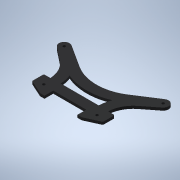
# Autodesk Inventor part: back_plate
Saved by Autodesk Inventor 2020 (Build 240168000, 168)
## iProperties
Created: 2016-01-08
Part Number: back_plate
Material: Genérico
Document SubType Name: Modeling
Designer: MIGUEL ANGEL
Density: 1 g/cm^3
Appearance: Goma - Negro
Author: MIGUEL ANGEL
Autodesk Inventor part; units mm, degrees
ref_plane "YZ Plane" through (0, 0, 0) normal (1, 0, 0) x (0, 1, 0)
ref_plane "XZ Plane" through (0, 0, 0) normal (0, 1, 0) x (-1, 0, 0)
sketch "Boceto1" plane through (0, 0, 0) normal (0, 0, 1) x (1, 0, 0)
  line L0 (20.4772, 24.8969) -> (57.9772, 24.8969)
  line L1 (86.0741, 43.5717) -> (86.0741, 43.5717)
  arc A0 (108.9954, 90.7434) -> (86.144, 46.4672) centre (146.0741, 43.5717) ccw
  arc A1 (20.4772, 85.7499) -> (75.1704, 101.8402) centre (20.4772, 186.7499) ccw
  line L2 (108.9954, 90.7434) -> (140.4433, 115.4625)
  arc A2 (140.4433, 115.4625) -> (125.6118, 134.3312) centre (133.0275, 124.8969) ccw
  line L3 (125.6118, 134.3312) -> (75.1704, 101.8402)
  line L4 (57.9772, 24.8969) -> (57.9772, 4.8969)
  line L5 (57.9772, 4.8969) -> (67.9772, 4.8969)
  line L6 (67.9772, 4.8969) -> (99.8761, 19.3004)
  line L7 (101.053, 21.1232) -> (101.053, 44.4672)
  line L8 (99.053, 46.4672) -> (86.144, 46.4672)
  line L9 (20.4772, -46.5022) -> (20.4772, 138.2428)
  arc A3 (101.053, 44.4672) -> (99.053, 46.4672) centre (99.053, 44.4672) ccw
  arc A4 (99.8761, 19.3004) -> (101.053, 21.1232) centre (99.053, 21.1232) ccw
  line L10 (20.4772, 24.8969) -> (-17.0228, 24.8969)
  line L11 (-45.1197, 43.5717) -> (-45.1197, 43.5717)
  arc A5 (-45.1896, 46.4672) -> (-68.041, 90.7434) centre (-105.1197, 43.5717) ccw
  arc A6 (-34.216, 101.8402) -> (20.4772, 85.7499) centre (20.4772, 186.7499) ccw
  line L12 (-68.041, 90.7434) -> (-99.4888, 115.4625)
  arc A7 (-84.6574, 134.3312) -> (-99.4888, 115.4625) centre (-92.0731, 124.8969) ccw
  line L13 (-84.6574, 134.3312) -> (-34.216, 101.8402)
  line L14 (-17.0228, 24.8969) -> (-17.0228, 4.8969)
  line L15 (-17.0228, 4.8969) -> (-27.0228, 4.8969)
  line L16 (-27.0228, 4.8969) -> (-58.9217, 19.3004)
  line L17 (-60.0986, 21.1232) -> (-60.0986, 44.4672)
  line L18 (-58.0986, 46.4672) -> (-45.1896, 46.4672)
  arc A8 (-58.0986, 46.4672) -> (-60.0986, 44.4672) centre (-58.0986, 44.4672) ccw
  arc A9 (-60.0986, 21.1232) -> (-58.9217, 19.3004) centre (-58.0986, 21.1232) ccw
  point P0 (0, 0)
  dimension "d0" = 37.5
  dimension "d1" = 60
  dimension "d3" = 40
  dimension "d4" = 12
  dimension "d5" = 60
  dimension "d6" = 101
  dimension "d7" = 2
  dimension "d21" = 10
  dimension "d23" = 35
  dimension "d42" = 100
  dimension "d43" = 20
  constraints: 38 end point, 20 point on circle, 17 symmetric about line, 10 centre point, 6 tangent, 4 point on line, 2 perpendicular, 2 vertical, 1 equal radius, 1 horizontal, 1 parallel, 1 vertical alignment, 5 other
  measures "d0" distance of L0.start L0.end
  measures "d1" radius of A0
  measures "d3" distance of L2.start L2.end
  measures "d4" radius of A2
  measures "d5" distance of L3.start L3.end
  measures "d6" radius of A1
  measures "d7" radius of A3
  measures "d21" distance of L4.end L5.end
  measures "d23" distance of L5.end L6.end
  measures "d42" distance from line of L0 A2.centre
  measures "d43" distance of L0.end L4.end
extrude "Extrusión1" add sketch "Boceto1" along normal blind 6
hole "Agujero1" at (-40.0986, 26.4672, 6) direction (0, 0, -1) diameter 6 end through all
ref_plane "Plano de trabajo1" through (20.4772, 21.1232, 0) normal (-1, 0, 0) x (0, 0, 1)
mirror "Simetría1" about plane through (20.4772, 21.1232, 0) normal (-1, 0, 0) of "Agujero1"
hole "Agujero2" at (-92.0731, 124.8969, 6) direction (0, 0, -1) diameter 6 end through all
hole "Agujero3" at (133.0275, 124.8969, 6) direction (0, 0, -1) diameter 6 end through all
sketch "Boceto3" plane through (0, 0, 6) normal (0, 0, 1) x (1, 0, 0)
  circle A0 centre (133.0275, 124.8969) radius 3 projected
  circle A1 centre (-92.0731, 124.8969) radius 3 projected
  circle A2 centre (81.053, 26.4672) radius 3 projected
  circle A3 centre (-40.0986, 26.4672) radius 3 projected
  arc A4 (-34.216, 101.8402) -> (75.1704, 101.8402) centre (20.4772, 186.7499) ccw projected
  line L0 (-34.216, 101.8402) -> (-84.6574, 134.3312) projected
  arc A5 (-84.6574, 134.3312) -> (-99.4888, 115.4625) centre (-92.0731, 124.8969) ccw projected
  line L1 (-99.4888, 115.4625) -> (-68.041, 90.7434) projected
  arc A6 (-45.1896, 46.4672) -> (-68.041, 90.7434) centre (-105.1197, 43.5717) ccw projected
  line L2 (-45.1896, 46.4672) -> (-58.0986, 46.4672) projected
  arc A7 (-58.0986, 46.4672) -> (-60.0986, 44.4672) centre (-58.0986, 44.4672) ccw projected
  line L3 (-60.0986, 44.4672) -> (-60.0986, 21.1232) projected
  arc A8 (-60.0986, 21.1232) -> (-58.9217, 19.3004) centre (-58.0986, 21.1232) ccw projected
  line L4 (-58.9217, 19.3004) -> (-27.0228, 4.8969) projected
  line L5 (-27.0228, 4.8969) -> (-17.0228, 4.8969) projected
  line L6 (-17.0228, 4.8969) -> (-17.0228, 24.8969) projected
  line L7 (-17.0228, 24.8969) -> (57.9772, 24.8969) projected
  line L8 (57.9772, 24.8969) -> (57.9772, 4.8969) projected
  line L9 (57.9772, 4.8969) -> (67.9772, 4.8969) projected
  line L10 (67.9772, 4.8969) -> (99.8761, 19.3004) projected
  arc A9 (99.8761, 19.3004) -> (101.053, 21.1232) centre (99.053, 21.1232) ccw projected
  line L11 (101.053, 21.1232) -> (101.053, 44.4672) projected
  arc A10 (101.053, 44.4672) -> (99.053, 46.4672) centre (99.053, 44.4672) ccw projected
  line L12 (99.053, 46.4672) -> (86.144, 46.4672) projected
  arc A11 (108.9954, 90.7434) -> (86.144, 46.4672) centre (146.0741, 43.5717) ccw projected
  line L13 (108.9954, 90.7434) -> (140.4433, 115.4625) projected
  arc A12 (140.4433, 115.4625) -> (125.6118, 134.3312) centre (133.0275, 124.8969) ccw projected
  line L14 (125.6118, 134.3312) -> (75.1704, 101.8402) projected
  arc A13 (-28.0705, 73.1557) -> (69.0249, 73.1557) centre (20.4772, 186.7499) ccw
  arc A14 (-22.6764, 47.4304) -> (-28.0705, 73.1557) centre (-105.1197, 43.5717) ccw
  line L15 (-22.6764, 47.4304) -> (63.6308, 47.4304)
  arc A15 (69.0249, 73.1557) -> (63.6308, 47.4304) centre (146.0741, 43.5717) ccw
  point P0 (0, 0)
  constraints: 6 point on circle, 3 centre point, 2 end point, 3 other
extrude "Extrusión3" cut sketch "Boceto3" against normal through all contours A13 A15 L15 A14
